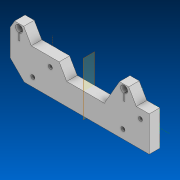
# Autodesk Inventor part: y-rear-VSLOT
Saved by Autodesk Inventor 2021 (Build 250183000, 183)
## iProperties
Created: 2021-03-08
Part Number: y-rear-VSLOT
Material: Generic
Document SubType Name: Modeling
Designer: Alex
Density: 1 g/cm^3
Appearance: Default
Author: Alex
## iProperties of the stored document _3DPrint.ipt
Created: 2021-03-08
Part Number: _3DPrint
Material: Generic
Document SubType Name: Modeling
Designer: Alex
Density: 1 g/cm^3
Appearance: Default
Author: Alex
Autodesk Inventor part; units mm, degrees
ref_plane "YZ Plane" through (0, 0, 0) normal (1, 0, 0) x (0, 1, 0)
ref_plane "XZ Plane" through (0, 0, 0) normal (0, 1, 0) x (-1, 0, 0)
ref_plane "XY Plane" through (0, 0, 0) normal (0, 0, 1) x (1, 0, 0)
sketch "rail_profile_1" plane through (0, 0, 0) normal (0, 0, 1) x (1, 0, 0)
  line L0 (6.605, 1.8) -> (6.605, 1.185) construction
  line L1 (7.1607, 6.1) -> (4.5, 3.4393) construction
  line L2 (4.5, 1.8) -> (6.605, 1.8) construction
  line L3 (4.5, 3.4393) -> (4.5, 1.8) construction
  line L4 (6.605, 1.185) -> (5.42, 0) construction
  line L5 (3.4393, 4.5) -> (6.1, 7.1607) construction
  line L6 (1.8, 4.5) -> (3.4393, 4.5) construction
  line L7 (1.8, 6.605) -> (1.8, 4.5) construction
  line L8 (5.42, 0) -> (1.5, 0) construction
  arc A0 (0, 1.5) -> (1.5, 0) centre (1.5, 1.5) ccw construction
  line L9 (0, 1.5) -> (0, 5.42) construction
  line L10 (0, 5.42) -> (1.185, 6.605) construction
  line L11 (1.185, 6.605) -> (1.8, 6.605) construction
  line L12 (0, 1.5) -> (0, 0) construction
  line L13 (0, 0) -> (1.5, 0) construction
  line L14 (3.7607, 17.3) -> (7.1607, 13.9) construction
  line L15 (1.8, 17.3) -> (3.7607, 17.3) construction
  line L16 (1.8, 22.7) -> (1.8, 17.3) construction
  line L17 (3.4393, 15.5) -> (1.8, 15.5) construction
  line L18 (1.8, 15.5) -> (1.8, 13.395) construction
  line L19 (1.8, 13.395) -> (1.185, 13.395) construction
  line L20 (6.1, 12.8393) -> (3.4393, 15.5) construction
  line L21 (1.185, 13.395) -> (0, 14.58) construction
  line L22 (0, 14.58) -> (0, 25.42) construction
  line L23 (6.1, 7.1607) -> (6.1, 9.79) construction
  line L24 (9.79, 6.1) -> (7.1607, 6.1) construction
  line L25 (6.1, 9.79) -> (6.31, 10) construction
  line L26 (10, 6.31) -> (9.79, 6.1) construction
  line L27 (6.31, 10) -> (6.1, 10.21) construction
  line L28 (10.21, 6.1) -> (10, 6.31) construction
  line L29 (6.1, 10.21) -> (6.1, 12.8393) construction
  circle A1 centre (10, 10) radius 2.3 construction
  line L30 (7.1607, 13.9) -> (12.8393, 13.9) construction
  line L31 (12.8393, 13.9) -> (13.9, 12.8393) construction
  line L32 (13.9, 12.8393) -> (13.9, 7.1607) construction
  line L33 (12.8393, 6.1) -> (10.21, 6.1) construction
  line L34 (17.3, 1.8) -> (22.7, 1.8) construction
  line L35 (17.3, 3.7607) -> (17.3, 1.8) construction
  line L36 (13.9, 7.1607) -> (17.3, 3.7607) construction
  line L37 (13.395, 1.185) -> (13.395, 1.8) construction
  line L38 (14.58, 0) -> (13.395, 1.185) construction
  line L39 (15.5, 3.4393) -> (12.8393, 6.1) construction
  line L40 (13.395, 1.8) -> (15.5, 1.8) construction
  line L41 (25.42, 0) -> (14.58, 0) construction
  line L42 (15.5, 1.8) -> (15.5, 3.4393) construction
  line L43 (0, 20) -> (51.5435, 20) construction
  line L44 (20, 0) -> (20, 50.2619) construction
  line L45 (33.395, 1.8) -> (33.395, 1.185) construction
  line L46 (32.8393, 6.1) -> (35.5, 3.4393) construction
  line L47 (35.5, 1.8) -> (33.395, 1.8) construction
  line L48 (35.5, 3.4393) -> (35.5, 1.8) construction
  line L49 (33.395, 1.185) -> (34.58, 0) construction
  line L50 (36.5607, 4.5) -> (33.9, 7.1607) construction
  line L51 (38.2, 4.5) -> (36.5607, 4.5) construction
  line L52 (38.2, 6.605) -> (38.2, 4.5) construction
  line L53 (34.58, 0) -> (38.5, 0) construction
  arc A2 (38.5, 0) -> (40, 1.5) centre (38.5, 1.5) ccw construction
  line L54 (40, 1.5) -> (40, 5.42) construction
  line L55 (38.815, 6.605) -> (38.2, 6.605) construction
  line L56 (40, 5.42) -> (38.815, 6.605) construction
  line L57 (33.9, 7.1607) -> (33.9, 9.79) construction
  line L58 (30.21, 6.1) -> (32.8393, 6.1) construction
  line L59 (33.9, 9.79) -> (33.69, 10) construction
  line L60 (30, 6.31) -> (30.21, 6.1) construction
  line L61 (33.69, 10) -> (33.9, 10.21) construction
  line L62 (29.79, 6.1) -> (30, 6.31) construction
  line L63 (33.9, 10.21) -> (33.9, 12.8393) construction
  line L64 (27.1607, 6.1) -> (29.79, 6.1) construction
  line L65 (26.1, 12.8393) -> (26.1, 7.1607) construction
  line L66 (32.8393, 13.9) -> (27.1607, 13.9) construction
  line L67 (27.1607, 13.9) -> (26.1, 12.8393) construction
  circle A3 centre (30, 10) radius 2.3 construction
  line L68 (38.2, 17.3) -> (36.2393, 17.3) construction
  line L69 (38.2, 22.7) -> (38.2, 17.3) construction
  line L70 (40, 14.58) -> (40, 25.42) construction
  line L71 (36.5607, 15.5) -> (38.2, 15.5) construction
  line L72 (38.2, 15.5) -> (38.2, 13.395) construction
  line L73 (38.2, 13.395) -> (38.815, 13.395) construction
  line L74 (38.815, 13.395) -> (40, 14.58) construction
  line L75 (22.7, 3.7607) -> (22.7, 1.8) construction
  line L76 (24.5, 1.8) -> (24.5, 3.4393) construction
  line L77 (26.605, 1.8) -> (24.5, 1.8) construction
  line L78 (26.605, 1.185) -> (26.605, 1.8) construction
  line L79 (25.42, 0) -> (26.605, 1.185) construction
  line L80 (24.5, 3.4393) -> (27.1607, 6.1) construction
  line L81 (26.1, 7.1607) -> (22.7, 3.7607) construction
  line L82 (33.9, 12.8393) -> (36.5607, 15.5) construction
  line L83 (36.2393, 17.3) -> (32.8393, 13.9) construction
  line L84 (6.605, 38.2) -> (6.605, 38.815) construction
  line L85 (7.1607, 33.9) -> (4.5, 36.5607) construction
  line L86 (4.5, 38.2) -> (6.605, 38.2) construction
  line L87 (4.5, 36.5607) -> (4.5, 38.2) construction
  line L88 (6.605, 38.815) -> (5.42, 40) construction
  line L89 (3.4393, 35.5) -> (6.1, 32.8393) construction
  line L90 (1.8, 35.5) -> (3.4393, 35.5) construction
  line L91 (1.8, 33.395) -> (1.8, 35.5) construction
  line L92 (5.42, 40) -> (1.5, 40) construction
  arc A4 (1.5, 40) -> (0, 38.5) centre (1.5, 38.5) ccw construction
  line L93 (0, 38.5) -> (0, 34.58) construction
  line L94 (1.185, 33.395) -> (1.8, 33.395) construction
  line L95 (0, 34.58) -> (1.185, 33.395) construction
  line L96 (6.1, 32.8393) -> (6.1, 30.21) construction
  line L97 (9.79, 33.9) -> (7.1607, 33.9) construction
  line L98 (6.1, 30.21) -> (6.31, 30) construction
  line L99 (10, 33.69) -> (9.79, 33.9) construction
  line L100 (6.31, 30) -> (6.1, 29.79) construction
  line L101 (10.21, 33.9) -> (10, 33.69) construction
  line L102 (6.1, 29.79) -> (6.1, 27.1607) construction
  line L103 (12.8393, 33.9) -> (10.21, 33.9) construction
  line L104 (13.9, 27.1607) -> (13.9, 32.8393) construction
  line L105 (7.1607, 26.1) -> (12.8393, 26.1) construction
  line L106 (12.8393, 26.1) -> (13.9, 27.1607) construction
  circle A5 centre (10, 30) radius 2.3 construction
  line L107 (1.8, 22.7) -> (3.7607, 22.7) construction
  line L108 (3.4393, 24.5) -> (1.8, 24.5) construction
  line L109 (1.8, 24.5) -> (1.8, 26.605) construction
  line L110 (1.8, 26.605) -> (1.185, 26.605) construction
  line L111 (1.185, 26.605) -> (0, 25.42) construction
  line L112 (17.3, 36.2393) -> (17.3, 38.2) construction
  line L113 (17.3, 38.2) -> (22.7, 38.2) construction
  line L114 (15.5, 38.2) -> (15.5, 36.5607) construction
  line L115 (13.395, 38.2) -> (15.5, 38.2) construction
  line L116 (13.395, 38.815) -> (13.395, 38.2) construction
  line L117 (14.58, 40) -> (13.395, 38.815) construction
  line L118 (25.42, 40) -> (14.58, 40) construction
  line L119 (15.5, 36.5607) -> (12.8393, 33.9) construction
  line L120 (13.9, 32.8393) -> (17.3, 36.2393) construction
  line L121 (6.1, 27.1607) -> (3.4393, 24.5) construction
  line L122 (3.7607, 22.7) -> (7.1607, 26.1) construction
  line L123 (38.815, 26.605) -> (40, 25.42) construction
  line L124 (38.2, 26.605) -> (38.815, 26.605) construction
  line L125 (38.2, 24.5) -> (38.2, 26.605) construction
  line L126 (38.2, 22.7) -> (36.2393, 22.7) construction
  line L127 (36.5607, 24.5) -> (38.2, 24.5) construction
  line L128 (36.2393, 22.7) -> (32.8393, 26.1) construction
  line L129 (33.9, 27.1607) -> (36.5607, 24.5) construction
  line L130 (32.8393, 26.1) -> (27.1607, 26.1) construction
  line L131 (27.1607, 26.1) -> (26.1, 27.1607) construction
  line L132 (26.1, 27.1607) -> (26.1, 32.8393) construction
  line L133 (26.1, 32.8393) -> (22.7, 36.2393) construction
  line L134 (24.5, 36.5607) -> (27.1607, 33.9) construction
  line L135 (24.5, 38.2) -> (24.5, 36.5607) construction
  line L136 (22.7, 36.2393) -> (22.7, 38.2) construction
  line L137 (26.605, 38.2) -> (24.5, 38.2) construction
  line L138 (26.605, 38.815) -> (26.605, 38.2) construction
  line L139 (25.42, 40) -> (26.605, 38.815) construction
  line L140 (33.395, 38.815) -> (34.58, 40) construction
  line L141 (34.58, 40) -> (38.5, 40) construction
  arc A6 (40, 38.5) -> (38.5, 40) centre (38.5, 38.5) ccw construction
  line L142 (40, 38.5) -> (40, 34.58) construction
  line L143 (40, 34.58) -> (38.815, 33.395) construction
  line L144 (38.815, 33.395) -> (38.2, 33.395) construction
  line L145 (38.2, 33.395) -> (38.2, 35.5) construction
  line L146 (38.2, 35.5) -> (36.5607, 35.5) construction
  line L147 (36.5607, 35.5) -> (33.9, 32.8393) construction
  line L148 (32.8393, 33.9) -> (35.5, 36.5607) construction
  line L149 (35.5, 36.5607) -> (35.5, 38.2) construction
  line L150 (35.5, 38.2) -> (33.395, 38.2) construction
  line L151 (33.395, 38.2) -> (33.395, 38.815) construction
  line L152 (30.21, 33.9) -> (32.8393, 33.9) construction
  line L153 (27.1607, 33.9) -> (29.79, 33.9) construction
  line L154 (30, 33.69) -> (30.21, 33.9) construction
  line L155 (29.79, 33.9) -> (30, 33.69) construction
  circle A7 centre (30, 30) radius 2.3 construction
  line L156 (33.9, 32.8393) -> (33.9, 30.21) construction
  line L157 (33.9, 30.21) -> (33.69, 30) construction
  line L158 (33.69, 30) -> (33.9, 29.79) construction
  line L159 (33.9, 29.79) -> (33.9, 27.1607) construction
  point P0 (0, 0)
  dimension "d0" = 1.5
  dimension "d1" = 6.605
  dimension "d2" = 6.605
  dimension "d3" = 1.185
  dimension "d4" = 135
  dimension "d5" = 1.185
  dimension "d6" = 135
  dimension "d7" = 0.615
  dimension "d8" = 0.615
  dimension "d9" = 2.105
  dimension "d10" = 1.6393
  dimension "d11" = 135
  dimension "d12" = 135
  dimension "d13" = 2.6607
  dimension "d14" = 1.6393
  dimension "d15" = 2.105
  dimension "d16" = 4.6
  dimension "d17" = 10
  dimension "d18" = 10
  dimension "d19" = 13.395
  dimension "d20" = 1.8
  dimension "d21" = 135
  dimension "d22" = 1.185
  dimension "d23" = 1.8
  dimension "d24" = 2.105
  dimension "d25" = 135
  dimension "d26" = 2.6607
  dimension "d29" = 7.1607
  dimension "d34" = 0.21
  dimension "d35" = 135
  dimension "d36" = 0.21
  dimension "d37" = 135
  dimension "d38" = 2.6293
  dimension "d39" = 3.4
  dimension "d40" = 1.5
  dimension "d41" = 135
  dimension "d42" = 0.21
  dimension "d43" = 0.21
  dimension "d44" = 135
  dimension "d45" = 2.6293
  dimension "d46" = 1.0607
  dimension "d47" = 135
  dimension "d48" = 5.6787
  dimension "d49" = 1.5
  dimension "d50" = 135
  dimension "d51" = 13.395
  dimension "d52" = 1.185
  dimension "d53" = 45
  dimension "d54" = 1.6393
  dimension "d55" = 1.9607
  dimension "d56" = 5.4
  dimension "d57" = 0.615
  dimension "d58" = 2.105
  dimension "d59" = 20
  dimension "d60" = 20
  constraints: 320 end point, 122 symmetric about line, 16 vertical, 13 horizontal, 8 centre point, 8 point on circle, 4 collinear, 2 midpoint, 2 parallel, 2 tangent, 1 coincident, 1 perpendicular, 6 other
  measures "d0" radius of A0
  measures "d1" distance between parallel lines of L0 L9
  measures "d2" distance between parallel lines of L11 L8
  measures "d3" horizontal distance of L9.end L11.start
  measures "d4" angle of L11 L10
  measures "d5" horizontal distance of L0.end L4.end
  measures "d6" angle of L0 L4
  measures "d7" distance of L11.start L7.start
  measures "d8" distance of L0.start L0.end
  measures "d9" distance of L7.start L6.start
  measures "d10" distance of L6.start L5.start
  measures "d11" angle of L5 L6
  measures "d12" angle of L1 L3
  measures "d13" horizontal distance of L5.start L5.end
  measures "d14" distance of L1.end L2.start
  measures "d15" distance of L2.start L0.start
  measures "d16" diameter of A1
  measures "d17" horizontal distance of A1.centre L12.end
  measures "d18" horizontal distance of point (0, 0) A1.centre
  measures "d19" distance from line of L37 point (0, 0)
  measures "d20" distance from line of L40 point (0, 0)
  measures "d21" angle of L41 L38
  measures "d22" horizontal distance of L38.start L37.start
  measures "d23" distance between parallel lines of L35 L42
  measures "d24" distance between parallel lines of L42 L37
  measures "d25" angle of L42 L39
  measures "d26" horizontal distance of L42.end L33.start
  measures "d29" horizontal distance of L1.start point (0, 0)
  measures "d34" horizontal distance of L26.start L24.start
  measures "d35" angle of L26 L24
  measures "d36" horizontal distance of L28.start L26.start
  measures "d37" angle of L33 L28
  measures "d38" distance of L24.start L1.start
  measures "d39" horizontal distance of L32.end L35.start
  measures "d40" distance between parallel lines of L36 L39
  measures "d41" angle of L25 L23
  measures "d42" horizontal distance of L23.end L25.end
  measures "d43" horizontal distance of L25.end L27.end
  measures "d44" angle of L29 L27
  measures "d45" distance of L5.end L23.end
  measures "d46" horizontal distance of L30.end L32.start
  measures "d47" angle of L32 L31
  measures "d48" distance of L30.start L30.end
  measures "d49" distance between parallel lines of L14 L20
  measures "d50" angle of L20 L29
  measures "d51" distance from line of point (0, 0) L19
  measures "d52" horizontal distance of L19.end L22.start
  measures "d53" angle of L19 L21
  measures "d54" distance of L17.start L17.end
  measures "d55" distance of L15.start L15.end
  measures "d56" distance of L16.start L15.start
  measures "d57" distance of L18.end L19.end
  measures "d58" distance of L17.end L18.end
  measures "d59" distance from line of L44 point (0, 0)
  measures "d60" distance from line of L43 L12.end
sketch "Sketch2" plane through (0, 0, 0) normal (0, 0, 1) x (1, 0, 0)
  line L0 (-14.2649, 439.4908) -> (-14.2649, -197.1126) construction
  line L1 (5.42, 40) -> (1.5, 40) construction
  line L2 (-119, 46.34) -> (-119, 16)
  line L3 (-114.0001, 55) -> (-119, 46.34)
  line L4 (-103.4701, 55) -> (-114.0001, 55)
  line L5 (-100.5834, 50) -> (-103.4701, 55)
  line L6 (3.1131, 50) -> (-100.5834, 50)
  line L7 (-119, 16) -> (-103, 0)
  line L8 (-103, 0) -> (40, 0)
  line L9 (5.9999, 55) -> (3.1131, 50)
  line L10 (16.5299, 55) -> (5.9999, 55)
  line L11 (25.1901, 40) -> (16.5299, 55)
  line L12 (40, 40) -> (25.1901, 40)
  line L13 (40, 0) -> (40, 40)
  circle A0 centre (-93, 10) radius 2.3
  circle A1 centre (-73, 30) radius 2.3
  line L14 (40, 14.58) -> (40, 25.42) construction
  circle A2 centre (10, 10) radius 2.3 projected
  circle A3 centre (30, 30) radius 2.3 projected
  line L15 (10, 10) -> (-93, 10) construction
  line L16 (25.42, 0) -> (14.58, 0) construction
  point P0 (0, 0)
  point P1 (0, 0)
  dimension "d219" = 20
  dimension "d220" = 20
  dimension "d221" = 120
  dimension "d222" = 83
  dimension "d223" = 60
  dimension "d224" = 60
  dimension "d225" = 120
  dimension "d226" = 10.53
  dimension "d227" = 10.53
  dimension "d228" = 4.0001
  dimension "d229" = 50
  dimension "d230" = 5
  dimension "d231" = 5
  dimension "d232" = 8.66
  dimension "d233" = 15
  dimension "d234" = 16
  dimension "d235" = 135
  dimension "d236" = 26
  constraints: 28 end point, 3 horizontal, 3 vertical, 2 centre point, 2 collinear, 2 equal radius
  measures "d219" horizontal distance of A1.centre L15.end
  measures "d220" horizontal distance of A1.centre L15.end
  measures "d221" angle of L4 L3
  measures "d222" horizontal distance of point (10, 10) A1.centre
  measures "d223" angle of L11 L10
  measures "d224" angle of L10 L9
  measures "d225" angle of L6 L5
  measures "d226" distance of L5.end L4.end
  measures "d227" distance of L10.start L9.start
  measures "d228" horizontal distance of L9.start point (10, 10)
  measures "d229" distance between parallel lines of L8 L6
  measures "d230" distance between parallel lines of L6 L10
  measures "d231" distance between parallel lines of L6 L4
  measures "d232" vertical distance of L4.end L2.start
  measures "d233" vertical distance of L11.start L10.start
  measures "d234" horizontal distance of L7.start L8.start
  measures "d235" angle of L8 L7
  measures "d236" distance from line of L2 L15.end
extrude "Base" add sketch "Sketch2" along normal blind 12
sketch "rail_profile_2" plane through (0, 0, 0) normal (0, 0, -1) x (-1, 0, 0)
  line L0 (-40, 38.5) -> (-40, 34.58) construction
  line L1 (-40, 34.58) -> (-38.815, 33.395) construction
  line L2 (0, 14.58) -> (0, 25.42) construction
  line L3 (69.605, 1.8) -> (69.605, 1.185) construction
  line L4 (70.1607, 6.1) -> (67.5, 3.4393) construction
  line L5 (67.5, 1.8) -> (69.605, 1.8) construction
  line L6 (67.5, 3.4393) -> (67.5, 1.8) construction
  line L7 (69.605, 1.185) -> (68.42, 0) construction
  line L8 (66.4393, 4.5) -> (69.1, 7.1607) construction
  line L9 (64.8, 4.5) -> (66.4393, 4.5) construction
  line L10 (64.8, 6.605) -> (64.8, 4.5) construction
  line L11 (68.42, 0) -> (64.5, 0) construction
  arc A0 (63, 1.5) -> (64.5, 0) centre (64.5, 1.5) ccw construction
  line L12 (63, 1.5) -> (63, 5.42) construction
  line L13 (64.185, 6.605) -> (64.8, 6.605) construction
  line L14 (63, 5.42) -> (64.185, 6.605) construction
  line L15 (63, 1.5) -> (63, 0) construction
  line L16 (63, 0) -> (64.5, 0) construction
  line L17 (69.1, 7.1607) -> (69.1, 9.79) construction
  line L18 (72.79, 6.1) -> (70.1607, 6.1) construction
  line L19 (69.1, 9.79) -> (69.31, 10) construction
  line L20 (73, 6.31) -> (72.79, 6.1) construction
  line L21 (69.31, 10) -> (69.1, 10.21) construction
  line L22 (73.21, 6.1) -> (73, 6.31) construction
  line L23 (69.1, 10.21) -> (69.1, 12.8393) construction
  line L24 (75.8393, 6.1) -> (73.21, 6.1) construction
  line L25 (76.9, 12.8393) -> (76.9, 7.1607) construction
  line L26 (70.1607, 13.9) -> (75.8393, 13.9) construction
  line L27 (75.8393, 13.9) -> (76.9, 12.8393) construction
  circle A1 centre (73, 10) radius 2.3 construction
  line L28 (64.8, 17.3) -> (66.7607, 17.3) construction
  line L29 (64.8, 22.7) -> (64.8, 17.3) construction
  line L30 (63, 14.58) -> (63, 25.42) construction
  line L31 (66.4393, 15.5) -> (64.8, 15.5) construction
  line L32 (64.8, 15.5) -> (64.8, 13.395) construction
  line L33 (64.8, 13.395) -> (64.185, 13.395) construction
  line L34 (64.185, 13.395) -> (63, 14.58) construction
  line L35 (80.3, 3.7607) -> (80.3, 1.8) construction
  line L36 (80.3, 1.8) -> (85.7, 1.8) construction
  line L37 (78.5, 1.8) -> (78.5, 3.4393) construction
  line L38 (76.395, 1.8) -> (78.5, 1.8) construction
  line L39 (76.395, 1.185) -> (76.395, 1.8) construction
  line L40 (77.58, 0) -> (76.395, 1.185) construction
  line L41 (88.42, 0) -> (77.58, 0) construction
  line L42 (78.5, 3.4393) -> (75.8393, 6.1) construction
  line L43 (76.9, 7.1607) -> (80.3, 3.7607) construction
  line L44 (69.1, 12.8393) -> (66.4393, 15.5) construction
  line L45 (66.7607, 17.3) -> (70.1607, 13.9) construction
  line L46 (63, 20) -> (44.0135, 20) construction
  line L47 (83, 0) -> (83, 50.2619) construction
  line L48 (103, 14.58) -> (103, 25.42) construction
  line L49 (101.815, 13.395) -> (103, 14.58) construction
  line L50 (101.2, 13.395) -> (101.815, 13.395) construction
  line L51 (101.2, 15.5) -> (101.2, 13.395) construction
  line L52 (101.2, 22.7) -> (101.2, 17.3) construction
  line L53 (101.2, 17.3) -> (99.2393, 17.3) construction
  line L54 (99.5607, 15.5) -> (101.2, 15.5) construction
  line L55 (99.2393, 17.3) -> (95.8393, 13.9) construction
  line L56 (96.9, 12.8393) -> (99.5607, 15.5) construction
  line L57 (95.8393, 13.9) -> (90.1607, 13.9) construction
  line L58 (90.1607, 13.9) -> (89.1, 12.8393) construction
  line L59 (89.1, 12.8393) -> (89.1, 7.1607) construction
  line L60 (89.1, 7.1607) -> (85.7, 3.7607) construction
  line L61 (87.5, 3.4393) -> (90.1607, 6.1) construction
  line L62 (87.5, 1.8) -> (87.5, 3.4393) construction
  line L63 (85.7, 3.7607) -> (85.7, 1.8) construction
  line L64 (89.605, 1.8) -> (87.5, 1.8) construction
  line L65 (89.605, 1.185) -> (89.605, 1.8) construction
  line L66 (88.42, 0) -> (89.605, 1.185) construction
  line L67 (96.395, 1.185) -> (97.58, 0) construction
  line L68 (97.58, 0) -> (101.5, 0) construction
  arc A2 (101.5, 0) -> (103, 1.5) centre (101.5, 1.5) ccw construction
  line L69 (103, 1.5) -> (103, 5.42) construction
  line L70 (103, 5.42) -> (101.815, 6.605) construction
  line L71 (101.815, 6.605) -> (101.2, 6.605) construction
  line L72 (101.2, 6.605) -> (101.2, 4.5) construction
  line L73 (101.2, 4.5) -> (99.5607, 4.5) construction
  line L74 (99.5607, 4.5) -> (96.9, 7.1607) construction
  line L75 (95.8393, 6.1) -> (98.5, 3.4393) construction
  line L76 (98.5, 3.4393) -> (98.5, 1.8) construction
  line L77 (98.5, 1.8) -> (96.395, 1.8) construction
  line L78 (96.395, 1.8) -> (96.395, 1.185) construction
  line L79 (93.21, 6.1) -> (95.8393, 6.1) construction
  line L80 (90.1607, 6.1) -> (92.79, 6.1) construction
  line L81 (93, 6.31) -> (93.21, 6.1) construction
  line L82 (92.79, 6.1) -> (93, 6.31) construction
  circle A3 centre (93, 10) radius 2.3 construction
  line L83 (96.9, 7.1607) -> (96.9, 9.79) construction
  line L84 (96.9, 9.79) -> (96.69, 10) construction
  line L85 (96.69, 10) -> (96.9, 10.21) construction
  line L86 (96.9, 10.21) -> (96.9, 12.8393) construction
  arc A4 (64.5, 40) -> (63, 38.5) centre (64.5, 38.5) ccw construction
  line L87 (68.42, 40) -> (64.5, 40) construction
  line L88 (69.605, 38.815) -> (68.42, 40) construction
  line L89 (69.605, 38.2) -> (69.605, 38.815) construction
  line L90 (67.5, 38.2) -> (69.605, 38.2) construction
  line L91 (67.5, 36.5607) -> (67.5, 38.2) construction
  line L92 (63, 38.5) -> (63, 34.58) construction
  line L93 (63, 34.58) -> (64.185, 33.395) construction
  line L94 (64.185, 33.395) -> (64.8, 33.395) construction
  line L95 (64.8, 33.395) -> (64.8, 35.5) construction
  line L96 (64.8, 35.5) -> (66.4393, 35.5) construction
  line L97 (66.4393, 35.5) -> (69.1, 32.8393) construction
  line L98 (70.1607, 33.9) -> (67.5, 36.5607) construction
  line L99 (72.79, 33.9) -> (70.1607, 33.9) construction
  line L100 (69.1, 32.8393) -> (69.1, 30.21) construction
  line L101 (73, 33.69) -> (72.79, 33.9) construction
  line L102 (73.21, 33.9) -> (73, 33.69) construction
  line L103 (75.8393, 33.9) -> (73.21, 33.9) construction
  circle A5 centre (73, 30) radius 2.3 construction
  line L104 (78.5, 36.5607) -> (75.8393, 33.9) construction
  line L105 (78.5, 38.2) -> (78.5, 36.5607) construction
  line L106 (76.395, 38.2) -> (78.5, 38.2) construction
  line L107 (76.395, 38.815) -> (76.395, 38.2) construction
  line L108 (77.58, 40) -> (76.395, 38.815) construction
  line L109 (88.42, 40) -> (77.58, 40) construction
  line L110 (80.3, 36.2393) -> (80.3, 38.2) construction
  line L111 (76.9, 32.8393) -> (80.3, 36.2393) construction
  line L112 (80.3, 38.2) -> (85.7, 38.2) construction
  line L113 (88.42, 40) -> (89.605, 38.815) construction
  line L114 (89.605, 38.815) -> (89.605, 38.2) construction
  line L115 (89.605, 38.2) -> (87.5, 38.2) construction
  line L116 (87.5, 38.2) -> (87.5, 36.5607) construction
  line L117 (85.7, 36.2393) -> (85.7, 38.2) construction
  line L118 (89.1, 32.8393) -> (85.7, 36.2393) construction
  line L119 (87.5, 36.5607) -> (90.1607, 33.9) construction
  line L120 (76.9, 27.1607) -> (76.9, 32.8393) construction
  line L121 (75.8393, 26.1) -> (76.9, 27.1607) construction
  line L122 (70.1607, 26.1) -> (75.8393, 26.1) construction
  line L123 (66.7607, 22.7) -> (70.1607, 26.1) construction
  line L124 (69.1, 29.79) -> (69.1, 27.1607) construction
  line L125 (69.1, 30.21) -> (69.31, 30) construction
  line L126 (69.31, 30) -> (69.1, 29.79) construction
  line L127 (66.4393, 24.5) -> (64.8, 24.5) construction
  line L128 (69.1, 27.1607) -> (66.4393, 24.5) construction
  line L129 (64.8, 22.7) -> (66.7607, 22.7) construction
  line L130 (64.8, 24.5) -> (64.8, 26.605) construction
  line L131 (64.8, 26.605) -> (64.185, 26.605) construction
  line L132 (64.185, 26.605) -> (63, 25.42) construction
  line L133 (90.1607, 33.9) -> (92.79, 33.9) construction
  line L134 (89.1, 27.1607) -> (89.1, 32.8393) construction
  line L135 (90.1607, 26.1) -> (89.1, 27.1607) construction
  line L136 (95.8393, 26.1) -> (90.1607, 26.1) construction
  line L137 (96.9, 29.79) -> (96.9, 27.1607) construction
  line L138 (99.2393, 22.7) -> (95.8393, 26.1) construction
  line L139 (99.5607, 24.5) -> (101.2, 24.5) construction
  line L140 (101.2, 22.7) -> (99.2393, 22.7) construction
  line L141 (96.9, 27.1607) -> (99.5607, 24.5) construction
  line L142 (101.2, 24.5) -> (101.2, 26.605) construction
  line L143 (101.2, 26.605) -> (101.815, 26.605) construction
  line L144 (101.815, 26.605) -> (103, 25.42) construction
  line L145 (103, 34.58) -> (101.815, 33.395) construction
  line L146 (103, 38.5) -> (103, 34.58) construction
  arc A6 (103, 38.5) -> (101.5, 40) centre (101.5, 38.5) ccw construction
  line L147 (97.58, 40) -> (101.5, 40) construction
  line L148 (96.395, 38.815) -> (97.58, 40) construction
  line L149 (96.395, 38.2) -> (96.395, 38.815) construction
  line L150 (98.5, 38.2) -> (96.395, 38.2) construction
  line L151 (93.21, 33.9) -> (95.8393, 33.9) construction
  line L152 (95.8393, 33.9) -> (98.5, 36.5607) construction
  line L153 (98.5, 36.5607) -> (98.5, 38.2) construction
  line L154 (99.5607, 35.5) -> (96.9, 32.8393) construction
  line L155 (96.9, 32.8393) -> (96.9, 30.21) construction
  line L156 (101.2, 35.5) -> (99.5607, 35.5) construction
  line L157 (101.2, 33.395) -> (101.2, 35.5) construction
  line L158 (101.815, 33.395) -> (101.2, 33.395) construction
  line L159 (96.9, 30.21) -> (96.69, 30) construction
  line L160 (96.69, 30) -> (96.9, 29.79) construction
  line L161 (93, 33.69) -> (93.21, 33.9) construction
  line L162 (92.79, 33.9) -> (93, 33.69) construction
  circle A7 centre (93, 30) radius 2.3 construction
  circle A8 centre (73, 30) radius 2.3 projected
  point P0 (0, 0)
  point P1 (93.2635, 30)
  dimension "d89" = 1.5
  dimension "d90" = 6.605
  dimension "d91" = 6.605
  dimension "d92" = 1.185
  dimension "d93" = 135
  dimension "d94" = 1.185
  dimension "d95" = 135
  dimension "d96" = 0.615
  dimension "d97" = 0.615
  dimension "d98" = 2.105
  dimension "d99" = 1.6393
  dimension "d100" = 135
  dimension "d101" = 135
  dimension "d102" = 2.6607
  dimension "d103" = 1.6393
  dimension "d104" = 2.105
  dimension "d105" = 4.6
  dimension "d106" = 10
  dimension "d107" = 10
  dimension "d108" = 13.395
  dimension "d109" = 1.8
  dimension "d110" = 135
  dimension "d111" = 1.185
  dimension "d112" = 1.8
  dimension "d113" = 2.105
  dimension "d114" = 135
  dimension "d115" = 2.6607
  dimension "d116" = 7.1607
  dimension "d117" = 0.21
  dimension "d118" = 135
  dimension "d119" = 0.21
  dimension "d120" = 135
  dimension "d121" = 2.6293
  dimension "d122" = 3.4
  dimension "d123" = 1.5
  dimension "d124" = 135
  dimension "d125" = 0.21
  dimension "d126" = 0.21
  dimension "d127" = 135
  dimension "d128" = 2.6293
  dimension "d129" = 1.0607
  dimension "d130" = 135
  dimension "d131" = 5.6787
  dimension "d132" = 1.5
  dimension "d133" = 135
  dimension "d134" = 13.395
  dimension "d135" = 1.185
  dimension "d136" = 45
  dimension "d137" = 1.6393
  dimension "d138" = 1.9607
  dimension "d139" = 5.4
  dimension "d140" = 0.615
  dimension "d141" = 2.105
  dimension "d142" = 20
  dimension "d143" = 20
  constraints: 320 end point, 42 symmetric about line, 16 vertical, 13 horizontal, 8 point on circle, 7 centre point, 4 collinear, 2 parallel, 2 tangent, 1 coincident, 1 midpoint, 1 perpendicular, 4 other
  measures "d89" radius of A0
  measures "d90" distance between parallel lines of L3 L12
  measures "d91" distance between parallel lines of L13 L11
  measures "d92" horizontal distance of L14.start L13.start
  measures "d93" angle of L13 L14
  measures "d94" horizontal distance of L7.start L11.start
  measures "d95" angle of L3 L7
  measures "d96" distance of L13.start L13.end
  measures "d97" distance of L3.start L7.start
  measures "d98" distance of L13.end L9.start
  measures "d99" distance of L9.start L9.end
  measures "d100" angle of L8 L9
  measures "d101" angle of L4 L6
  measures "d102" horizontal distance of L9.end L17.start
  measures "d103" distance of L6.start L6.end
  measures "d104" distance of L6.end L3.start
  measures "d105" diameter of A1
  measures "d106" horizontal distance of A1.centre L16.start
  measures "d107" horizontal distance of point (63, 0) A1.centre
  measures "d108" distance from line of L39 point (63, 0)
  measures "d109" distance from line of L38 point (63, 0)
  measures "d110" angle of L41 L40
  measures "d111" horizontal distance of L41.end L39.start
  measures "d112" distance between parallel lines of L35 L37
  measures "d113" distance between parallel lines of L37 L39
  measures "d114" angle of L37 L42
  measures "d115" horizontal distance of L37.end L42.end
  measures "d116" horizontal distance of L18.end point (63, 0)
  measures "d117" horizontal distance of L20.start L18.start
  measures "d118" angle of L20 L18
  measures "d119" horizontal distance of L22.start L20.start
  measures "d120" angle of L24 L22
  measures "d121" distance of L18.start L18.end
  measures "d122" horizontal distance of L25.end L35.start
  measures "d123" distance between parallel lines of L43 L42
  measures "d124" angle of L19 L17
  measures "d125" horizontal distance of L19.start L21.start
  measures "d126" horizontal distance of L21.start L23.start
  measures "d127" angle of L23 L21
  measures "d128" distance of L17.start L19.start
  measures "d129" horizontal distance of L26.end L25.start
  measures "d130" angle of L25 L27
  measures "d131" distance of L45.end L26.end
  measures "d132" distance between parallel lines of L45 L44
  measures "d133" angle of L44 L23
  measures "d134" distance from line of point (63, 0) L33
  measures "d135" horizontal distance of L33.end L34.end
  measures "d136" angle of L33 L34
  measures "d137" distance of L44.end L31.end
  measures "d138" distance of L29.end L45.start
  measures "d139" distance of L29.start L29.end
  measures "d140" distance of L33.start L33.end
  measures "d141" distance of L31.end L33.start
  measures "d142" distance from line of L47 point (63, 0)
  measures "d143" distance from line of L46 L16.start
sketch "Sketch3" plane through (0, 0, 12) normal (0, 0, 1) x (1, 0, 0)
  arc A0 (11.6399, 45.9423) -> (10.8899, 45.9423) centre (11.2649, 50) ccw
  line L0 (11.2649, 55) -> (11.2649, 50) construction
  line L1 (10.8899, 45.9423) -> (10.8899, 37.9423)
  line L2 (11.6399, 45.9423) -> (11.6399, 37.9423)
  line L3 (10.8899, 37.9423) -> (11.6399, 37.9423)
  line L4 (-48.7351, 50) -> (-48.7351, 99.3964) construction
  arc A1 (-108.3601, 45.9423) -> (-109.1101, 45.9423) centre (-108.7351, 50) ccw
  line L5 (-108.3601, 45.9423) -> (-108.3601, 37.9423)
  line L6 (-109.1101, 45.9423) -> (-109.1101, 37.9423)
  line L7 (-108.3601, 37.9423) -> (-109.1101, 37.9423)
  line L8 (16.5299, 55) -> (5.9999, 55) construction
  line L9 (11.2649, 55) -> (11.2649, 50) construction
  point P0 (0, 0)
  dimension "d83" = 5
  dimension "d84" = 8.15
  dimension "d85" = 8
  dimension "d86" = 0.75
  dimension "d237" = 120
  constraints: 18 end point, 6 symmetric about line, 4 point on circle, 4 vertical, 2 centre point, 2 coincident, 2 midpoint, 1 horizontal, 1 parallel, 2 other
  measures "d83" distance of L0.end L0.start
  measures "d84" diameter of A0
  measures "d85" distance of L2.start L2.end
  measures "d86" distance of L1.end L2.end
  measures "d237" distance of A0.centre A1.centre
extrude "rod_holes" cut sketch "Sketch3" against normal blind 10
ref_plane "Work Plane2" through (-35, 0, 12) normal (1, 0, 0) x (0, 0, -1)
ref_plane "Work Plane1" through (40, 0, 12) normal (1, 0, 0) x (0, 0, -1)
sketch "Sketch14" plane through (0, 0, 12) normal (0, 0, 1) x (1, 0, 0)
  line L0 (3.1131, 50) -> (-100.5834, 50) projected
  line L1 (-100.5834, 50) -> (-94.8099, 40)
  line L2 (-94.8099, 40) -> (-2.6604, 40)
  line L3 (-2.6604, 40) -> (3.1131, 50)
  line L4 (5.9999, 55) -> (3.1131, 50) projected
  line L5 (-100.5834, 50) -> (-103.4701, 55) projected
  line L6 (-103, 0) -> (40, 0) projected
  line L7 (-63, 40) -> (-54.3397, 25)
  line L8 (-54.3397, 25) -> (-11.3207, 25)
  circle A0 centre (-73, 30) radius 2.3 projected
  line L9 (-2.6604, 40) -> (-11.3207, 25)
  line L10 (-103, 0) -> (-63, 0) construction
  line L11 (-63, 0) -> (-63, 40) construction
  line L12 (-63, 40) -> (-103, 40) construction
  line L13 (-103, 40) -> (-103, 0) construction
  circle A1 centre (-93, 10) radius 2.3 projected
  line L14 (40, 0) -> (0, 0) construction
  line L15 (0, 0) -> (0, 40) construction
  line L16 (0, 40) -> (40, 40) construction
  line L17 (40, 40) -> (40, 0) construction
  circle A2 centre (30, 30) radius 2.3 projected
  point P0 (0, 0)
  dimension "d283" = 40
  dimension "d284" = 10
  dimension "d285" = 15
  dimension "d286" = 40
  dimension "d287" = 40
  dimension "d288" = 10
  dimension "d289" = 40
  dimension "d290" = 40
  dimension "d291" = 10
  constraints: 28 end point, 5 collinear, 5 parallel, 4 horizontal, 2 perpendicular, 1 point on line
  measures "d283" distance between parallel lines of L2 L6
  measures "d284" horizontal distance of A0.centre L7.start
  measures "d285" distance between parallel lines of L2 L8
  measures "d286" distance of L11.end L12.end
  measures "d287" distance of L10.end L11.end
  measures "d288" distance from line of L13 A1.centre
  measures "d289" distance of L16.end L14.start
  measures "d290" distance of L15.end L16.end
  measures "d291" distance from line of L17 A2.centre
extrude "Extrusion11" cut sketch "Sketch14" against normal through all contours L3 L2 L1 L0 | L9 L8 L7 L2
body "Solid1"
